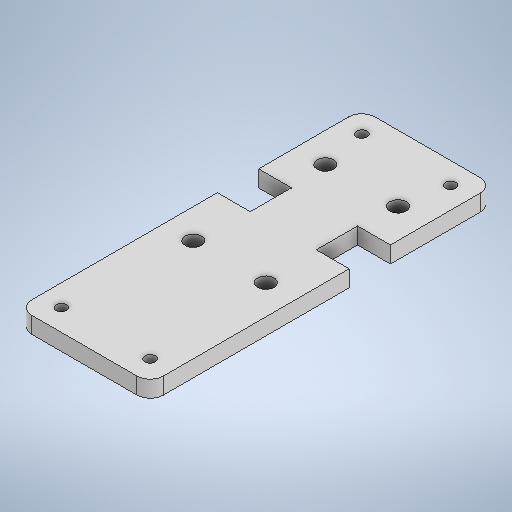
# Autodesk Inventor part: bottom
Saved by Autodesk Inventor 2025.2 (Build 292293000, 293)
## iProperties
Created: 2025-02-15
Part Number: bottom
Material: Generic
Document SubType Name: Modeling
Designer: Admin
Density: 1 g/cm^3
Appearance: Default
Author: Admin
Autodesk Inventor part; units mm, degrees
ref_plane "YZ Plane" through (0, 0, 0) normal (1, 0, 0) x (0, 1, 0)
ref_plane "XZ Plane" through (0, 0, 0) normal (0, 1, 0) x (-1, 0, 0)
ref_plane "XY Plane" through (0, 0, 0) normal (0, 0, 1) x (1, 0, 0)
sketch "Sketch1" plane through (0, 0, 0) normal (0, 1, 0) x (-1, 0, 0)
  point P0 (0, 0)
sketch "Sketch2" plane through (0, 0, 0) normal (0, 1, 0) x (-1, 0, 0)
  line L0 (-19.9525, 52) -> (19.9525, 52)
  line L1 (19.9525, 52) -> (19.9525, -52)
  line L2 (19.9525, -52) -> (-19.9525, -52)
  line L3 (-19.9525, -52) -> (-19.9525, 52)
  line L4 (-19.9525, 52) -> (19.9525, -52) construction
  line L5 (19.9525, 52) -> (-19.9525, -52) construction
  circle A0 centre (13.4525, 45.5) radius 1.6
  circle A1 centre (-13.4525, 45.5) radius 1.6
  line L6 (0, 59.3125) -> (0, -64.5558)
  line L7 (36.5125, 0) -> (-39.6875, 0)
  circle A2 centre (13.4525, -45.5) radius 1.6
  circle A3 centre (-13.4525, -45.5) radius 1.6
  line L8 (0, -59.3125) -> (0, 64.5558)
  circle A4 centre (11, 8) radius 2.5
  circle A5 centre (-11, 8) radius 2.5
  circle A6 centre (-11, -32) radius 2.5
  circle A7 centre (11, -32) radius 2.5
  line L9 (-10, -8.25) -> (-19, -8.25)
  line L10 (-19, -20.75) -> (-10, -20.75)
  line L11 (-10, -20.75) -> (-10, -8.25)
  line L12 (-10, -8.25) -> (-19, -20.75) construction
  line L13 (-19, -8.25) -> (-10, -20.75) construction
  line L14 (-10, -8.25) -> (-19.9525, -8.25)
  line L15 (-19.9525, -8.25) -> (-19.9525, -20.75)
  line L16 (-19.9525, -20.75) -> (-10, -20.75)
  line L17 (-10, -20.75) -> (-10, -8.25)
  line L18 (10, -8.25) -> (19, -8.25)
  line L19 (19, -20.75) -> (10, -20.75)
  line L20 (10, -20.75) -> (10, -8.25)
  line L21 (10, -8.25) -> (19, -20.75) construction
  line L22 (19, -8.25) -> (10, -20.75) construction
  line L23 (10, -8.25) -> (19.9525, -8.25)
  line L24 (19.9525, -8.25) -> (19.9525, -20.75)
  line L25 (19.9525, -20.75) -> (10, -20.75)
  line L26 (10, -20.75) -> (10, -8.25)
  point P0 (0, 0)
  point P1 (-14.5, -14.5)
  point P2 (14.5, -14.5)
  dimension "d0" = 104
  dimension "d1" = 39.905
  dimension "d2" = 3.2
  dimension "d3" = 3.2
  dimension "d5" = 6.5
  dimension "d7" = 6.5
  dimension "d11" = 5
  dimension "d12" = 5
  dimension "d13" = 11
  dimension "d14" = 11
  dimension "d15" = 8
  dimension "d16" = 8
  dimension "d17" = 5
  dimension "d18" = 5
  dimension "d19" = 40
  dimension "d20" = 40
  dimension "d21" = 11
  dimension "d22" = 11
  dimension "d23" = 12.5
  dimension "d24" = 9
  dimension "d25" = 8.25
  dimension "d26" = 10
  dimension "d27" = 6.5
  dimension "d28" = 6.5
  constraints: 54 end point, 12 symmetric about line, 8 centre point, 5 parallel, 4 horizontal, 4 midpoint, 3 point on line, 2 perpendicular, 1 vertical, 2 other
  measures "d0" distance of L0.end L1.end
  measures "d1" distance of L1.end L2.end
  measures "d2" diameter of A0
  measures "d3" diameter of A1
  measures "d5" distance from line of L0 A0.centre
  measures "d7" distance from line of L0 A1.centre
  measures "d11" diameter of A4
  measures "d12" diameter of A5
  measures "d13" distance from line of L6 A4.centre
  measures "d14" distance from line of L8 A5.centre
  measures "d15" distance from line of L7 A5.centre
  measures "d16" distance from line of L7 A4.centre
  measures "d17" diameter of A6
  measures "d18" diameter of A7
  measures "d19" distance of A7.centre A4.centre
  measures "d20" distance of A5.centre A6.centre
  measures "d21" distance from line of L6 A7.centre
  measures "d22" distance from line of L6 A6.centre
  measures "d23" distance of L10.end L9.start
  measures "d24" distance of L10.start L10.end
  measures "d25" distance between parallel lines of L7 L9
  measures "d26" distance between parallel lines of L8 L11
  measures "d27" distance from line of L3 A1.centre
  measures "d28" distance from line of L1 A0.centre
extrude "Extrusion1" add sketch "Sketch2" along normal blind 5 contours L0 L6 L7 L3 | L0 L1 L7 L6 | L7 L6 L2 L3 L16 L10 L11 L9 L14 | L7 L1 L23 L18 L20 L19 L25 L2 L6
fillet "Fillet1" radius 4 4 edges at (19.9525, 2.5, 52) (-19.9525, 2.5, 52) (19.9525, 2.5, -52) (-19.9525, 2.5, -52)
body "Solid1"
